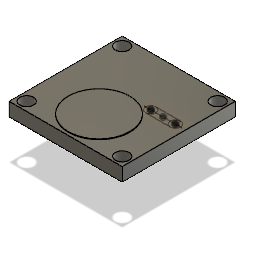
Capacitative Touch Sensor TTP223B v2 (Autodesk Fusion 360 design; units mm, degrees)
Autodesk Fusion 360 part; units mm, degrees
note: some values were not read from the file. Set by a fixed rule: which sketch regions a step uses.
sketch "Sketch1" plane through (0, 0, 0) normal (0, 1, 0) x (1, 0, 0)
  line L0 (0, 0) -> (16.6, 0)
  line L1 (16.6, 0) -> (16.6, -16.6)
  line L2 (16.6, -16.6) -> (0, -16.6)
  line L3 (0, -16.6) -> (0, 0)
  line L4 (16.6, -16.6) -> (8.3, -16.6)
  line L5 (8.3, -16.6) -> (8.3, -11.7) construction
  circle A0 centre (8.3, -11.7) radius 4.5
  line L6 (16.6, -16.6) -> (15.3, -16.6)
  line L7 (16.6, -16.6) -> (16.6, -15.3)
  line L8 (15.3, -16.6) -> (15.3, -14) construction
  line L9 (16.6, -15.3) -> (14, -15.3) construction
  circle A1 centre (15.3, -15.3) radius 1
  circle A2 centre (1.3, -15.3) radius 1
  line L10 (0, -8.3) -> (16.6, -8.3) construction
  circle A3 centre (15.3, -1.3) radius 1
  circle A4 centre (1.3, -1.3) radius 1
  line L11 (8.3, 0) -> (8.3, -3.6)
  line L12 (5.5, -1) -> (11.1, -1)
  line L13 (11.1, -1) -> (11.1, -3.6)
  line L14 (11.1, -3.6) -> (5.5, -3.6)
  line L15 (5.5, -3.6) -> (5.5, -1)
  line L16 (13.6, 0) -> (13.6, -5.6) construction
  line L17 (16.6, -5.8) -> (13.6, -5.8) construction
  line L18 (14.6, -2.8) -> (12.6, -2.8)
  line L19 (12.6, -2.8) -> (12.6, -5.8)
  line L20 (12.6, -5.8) -> (14.6, -5.8)
  line L21 (14.6, -5.8) -> (14.6, -2.8)
  line L22 (3.0224, 0) -> (3.0224, -2.2) construction
  line L23 (0, -2.5501) -> (2.6, -2.5501) construction
  line L24 (2.6, -2.2) -> (4.9, -2.2)
  line L25 (4.9, -2.2) -> (4.9, -3.6)
  line L26 (4.9, -3.6) -> (2.6, -3.6)
  line L27 (2.6, -3.6) -> (2.6, -2.2)
  line L28 (0, -5.4812) -> (1.5, -5.4812) construction
  line L29 (2, 0) -> (2, -4) construction
  line L30 (1.5, -4) -> (3, -4)
  line L31 (3, -4) -> (3, -6.4)
  line L32 (3, -6.4) -> (1.5, -6.4)
  line L33 (1.5, -6.4) -> (1.5, -4)
  line L34 (3.1, -4) -> (4.6, -4)
  line L35 (4.6, -4) -> (4.6, -6.4)
  line L36 (4.6, -6.4) -> (3.1, -6.4)
  line L37 (3.1, -6.4) -> (3.1, -4)
  line L38 (0, -6) -> (3.1, -6) construction
  line L39 (12.35, -5.95) -> (14.85, -5.95)
  line L40 (14.85, -5.95) -> (14.85, -7.45)
  line L41 (14.85, -7.45) -> (12.35, -7.45)
  line L42 (12.35, -7.45) -> (12.35, -5.95)
  line L43 (13.6, -5.8) -> (13.6, -5.95)
  dimension "d1" = 16.6
  dimension "d2" = 16.6
  dimension "d3" = 8.3
  dimension "d4" = 4.9
  dimension "d5" = 9
  dimension "d6" = 1.3
  dimension "d7" = 1.3
  dimension "d8" = 2
  dimension "d9" = 3.6
  dimension "d10" = 5.6
  dimension "d11" = 2.6
  dimension "d12" = 5.6
  dimension "d13" = 3
  dimension "d14" = 2
  dimension "d15" = 3
  dimension "d16" = 2.8
  dimension "d17" = 2.2
  dimension "d18" = 2.6
  dimension "d19" = 2.3
  dimension "d20" = 1.4
  dimension "d21" = 1.5
  dimension "d22" = 4
  dimension "d23" = 1.5
  dimension "d24" = 2.4
  dimension "d25" = 1.5
  dimension "d26" = 2.4
  dimension "d27" = 3.1
  dimension "d28" = 2.5
  dimension "d29" = 1.5
  dimension "d30" = 0.15
  constraint horizontal L0
  constraint vertical L1
  constraint horizontal L2
  constraint vertical L3
  constraint coincident L0.start L3.end
  constraint midpoint L2 L4.end
  constraint perpendicular L2 L5
  constraint coincident L5.end A0.centre
  constraint perpendicular L1 L6
  constraint perpendicular L6 L7
  constraint perpendicular L6 L8
  constraint perpendicular L8 L9
  constraint midpoint L9 A1.centre
  constraint symmetric L5 A1 A2
  constraint midpoint L3 L10.start
  constraint midpoint L1 L10.end
  constraint symmetric A1 L10 A3
  constraint symmetric A2 L10 A4
  constraint midpoint L0 L11.start
  constraint perpendicular L0 L11
  constraint horizontal L12
  constraint vertical L13
  constraint horizontal L14
  constraint vertical L15
  constraint coincident L11.end L14
  constraint symmetric L11 L13 L15
  constraint coincident L0 L16.start
  constraint perpendicular L12 L16
  constraint coincident L1 L17.start
  constraint perpendicular L16 L17
  constraint coincident L16 L17.end
  constraint horizontal L18
  constraint vertical L19
  constraint horizontal L20
  constraint vertical L21
  constraint coincident L17.end L20
  constraint symmetric L16 L19 L21
  constraint coincident L0 L22.start
  constraint perpendicular L0 L22
  constraint coincident L3 L23.start
  constraint perpendicular L3 L23
  constraint horizontal L24
  constraint vertical L25
  constraint horizontal L26
  constraint vertical L27
  constraint coincident L22.end L24
  constraint coincident L23.end L27
  constraint coincident L3 L28.start
  constraint perpendicular L3 L28
  constraint coincident L0 L29.start
  constraint perpendicular L23 L29
  constraint horizontal L30
  constraint vertical L31
  constraint horizontal L32
  constraint vertical L33
  constraint horizontal L34
  constraint vertical L35
  constraint horizontal L36
  constraint vertical L37
  constraint coincident L3 L38.start
  constraint perpendicular L3 L38
  constraint coincident L28.end L33
  constraint coincident L29.end L30
  constraint coincident L37 L38.end
  constraint coincident L29.end L34
  constraint horizontal L39
  constraint vertical L40
  constraint horizontal L41
  constraint vertical L42
  constraint vertical L43
  constraint coincident L39 L43.end
  constraint symmetric L16 L40 L42
  measures "d1" distance of L0.start L0.end
  measures "d2" distance of L0.start L2.end
  measures "d3" distance of L1.end L4.end
  measures "d4" distance of L4.end L5.end
  measures "d5" diameter of A0
  measures "d6" distance of L1.end L6.end
  measures "d7" distance of L1.end L7.end
  measures "d8" diameter of A1
  measures "d9" distance of L11.start L11.end
  measures "d10" distance of L12.start L12.end
  measures "d11" distance of L12.start L14.end
  measures "d12" distance of L16.start L16.end
  measures "d13" distance of L17.start L17.end
  measures "d14" distance of L18.start L18.end
  measures "d15" distance of L17 L18
  measures "d16" distance of L0 L18
  measures "d17" distance of L22.start L22.end
  measures "d18" distance of L23.start L23.end
  measures "d19" distance of L24.start L24.end
  measures "d20" distance of L24.start L26.end
  measures "d21" distance of L28.start L28.end
  measures "d22" distance of L29.start L29.end
  measures "d23" distance of L30.start L30.end
  measures "d24" distance of L30.start L32.end
  measures "d25" distance of L34.start L34.end
  measures "d26" distance of L34.start L36.end
  measures "d27" distance of L38.start L38.end
  measures "d28" distance of L39.start L39.end
  measures "d29" distance of L39.start L41.end
  measures "d30" distance of L17.end L43.end
extrude "Extrude1" add sketch "Sketch1" along normal blind 2 contours L0 L1 L2 L3 L4 L6 L7 | A0 | L11 L12 L13 L14 | L11 L12 L14 L15 | L18 L19 L20 L21 | L24 L25 L26 L27 | L30 L31 L32 L33 | L34 L35 L36 L37 | L39 L40 L41 L42 makes body 1
extrude "Extrude2" add sketch "Sketch1" along normal blind 2.1 contours A0 bodies 1
extrude "Extrude3" cut sketch "Sketch1" along normal blind 0.05 contours A0 bodies 1
extrude "Extrude4" add sketch "Sketch1" against normal blind 0.5 contours L18 L19 L20 L21 | L24 L25 L26 L27 | L30 L31 L32 L33 | L34 L35 L36 L37 | L39 L40 L41 L42 bodies 1
extrude "Extrude5" add sketch "Sketch1" against normal blind 3 contours L11 L12 L13 L14 | L11 L12 L14 L15 bodies 1
sketch "Sketch2" plane through (0, -3, 0) normal (0, -1, 0) x (1, 0, 0)
  line L0 (11.1, 3.6) -> (5.5, 3.6)
  line L1 (5.5, 3.6) -> (5.5, 1)
  line L2 (5.5, 1) -> (11.1, 1)
  line L3 (11.1, 1) -> (11.1, 3.6)
  line L4 (5.5, 2.3) -> (11.1, 2.3)
  circle A0 centre (8.3, 2.3) radius 0.25
  line L5 (5.5, 2.3) -> (6.5, 2.3)
  circle A1 centre (6.5, 2.3) radius 0.25
  line L6 (11.1, 2.3) -> (10.1, 2.3)
  circle A2 centre (10.1, 2.3) radius 0.25
  circle A3 centre (6.5, 2.3) radius 0.75
  circle A4 centre (10.1, 2.3) radius 0.75
  line L7 (10.1, 3.05) -> (6.5, 3.05)
  line L8 (10.1, 1.55) -> (6.5, 1.55)
  dimension "d41" = 0.5
  dimension "d42" = 1
  dimension "d43" = 0.5
  dimension "d44" = 1
  dimension "d45" = 0.5
  dimension "d46" = 1.5
  dimension "d47" = 1.5
  constraint midpoint L1 L4.start
  constraint midpoint L3 L4.end
  constraint midpoint L4 A0.centre
  constraint perpendicular L1 L5
  constraint coincident L5.end A1.centre
  constraint perpendicular L3 L6
  constraint coincident L6.end A2.centre
  constraint coincident A4 L7.start
  constraint tangent A4 L7
  constraint coincident A3 L7.end
  constraint tangent A3 L7
  constraint coincident A4 L8.start
  constraint tangent A4 L8
  constraint coincident A3 L8.end
  constraint tangent A3 L8
  measures "d41" diameter of A0
  measures "d42" distance of L4.start L5.end
  measures "d43" diameter of A1
  measures "d44" distance of L4.end L6.end
  measures "d45" diameter of A2
  measures "d46" diameter of A3
  measures "d47" diameter of A4
extrude "Extrude6" add sketch "Sketch2" along normal blind 3 separate body contours L4 L6 A2 A4 | L4 L6 A2 A4 | L4 L5 A1 A3 | L4 L5 A1 A3 | L4 A0 A3 A4 L7 | L4 A0 A3 A4 L8 makes body 2
extrude "Extrude7" add sketch "Sketch2" along normal blind 4.5 separate body contours L4 A0 A3 A4 L7 makes body 3
sketch "Sketch3" plane through (0, 0, 2.3) normal (0, 0, -1) x (-1, 0, 0)
  line L0 (-7.25, -3) -> (-8.05, -3)
  line L1 (-8.05, -3) -> (-8.05, -7.5)
  line L2 (-8.05, -7.5) -> (-7.25, -7.5)
  line L3 (-7.25, -7.5) -> (-7.25, -3)
  line L4 (-7.65, -7.5) -> (-8.3, -7.5)
  line L5 (-7.65, -7.5) -> (-6.5, -7.5)
  line L6 (-6.5, -7.5) -> (-6.5, -6.75)
  circle A0 centre (-6.5, -6.75) radius 0.75
  line L7 (-5.75, -6.75) -> (-5.75, -5.6822)
  line L8 (-5.75, -5.6822) -> (-6.7545, -6.0445)
  line L9 (-8.3, -7.5) -> (-10.1, -7.5)
  line L10 (-10.1, -7.5) -> (-10.1, -6.75)
  circle A1 centre (-10.1, -6.75) radius 0.75
  line L11 (-10.85, -6.75) -> (-10.85, -5.6967)
  line L12 (-10.85, -5.6967) -> (-9.8547, -6.0413)
  line L13 (-10.85, -5.6967) -> (-5.75, -5.6822)
  dimension "d52" = 0.65
  dimension "d53" = 1.15
  dimension "d54" = 0.75
  dimension "d55" = 1.5
  dimension "d56" = 1.8
  dimension "d57" = 0.75
  dimension "d58" = 1.5
  constraint midpoint L2 L4.start
  constraint perpendicular L1 L4
  constraint parallel L2 L5
  constraint perpendicular L5 L6
  constraint coincident L6.end A0.centre
  constraint coincident A0 L7.start
  constraint tangent A0 L7
  constraint vertical L7
  constraint coincident A0 L8.end
  constraint parallel L4 L9
  constraint perpendicular L9 L10
  constraint coincident L10.end A1.centre
  constraint coincident A1 L11.start
  constraint tangent A1 L11
  constraint perpendicular L9 L11
  constraint coincident A1 L12.end
  constraint tangent A1 L12
  constraint tangent A0 L8
  measures "d52" distance of L4.start L4.end
  measures "d53" distance of L4.start L5.end
  measures "d54" distance of L5.end L6.end
  measures "d55" diameter of A0
  measures "d56" distance of L4.end L9.end
  measures "d57" distance of L9.end L10.end
  measures "d58" diameter of A1
delete_body "RemoveBody1" bodies 3
extrude "Extrude8" add sketch "Sketch3" along normal blind -0.75 and the other way blind -4 separate body contours L3 A0 L8 L13 | L1 L2 L3 L4 L5 L13 | L1 L4 L9 A1 L12 L13 | L3 L5 A0 | A0 | A0 L7 L8 | A1 L11 L12 | A1 makes body 4
extrude "Extrude9" cut 1 faces at (8.3062, -6, 1.7169) along direction (0, 1, 0) blind 1.75 on bodies 2 bodies 2
extrude "Extrude10" cut sketch "Sketch2" against normal blind 0.5 contours L0 L1 L3 L4 L5 L6 A3 A4 L7 | L1 L2 L3 L4 L5 L6 A3 A4 L8 bodies 1
move_body "Move1" bodies 4 to x (1, 0, 0) y (0, 1, 0) z (0, 0, 1) at (0, 1.75, 0)
combine "Combine1" operation add target body 1 tool bodies 2 4
